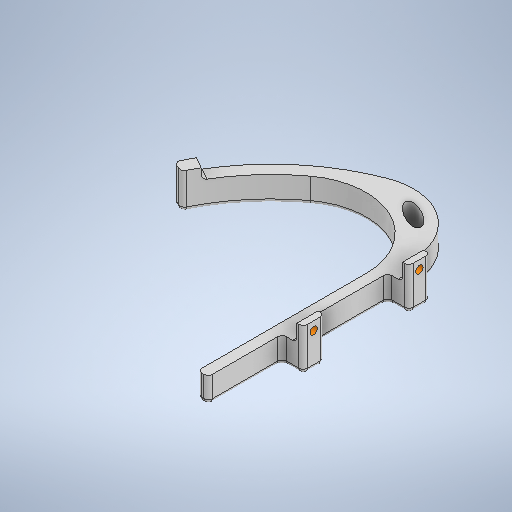
# Autodesk Inventor part: pare-chocs
Saved by Autodesk Inventor 2025 (Build 290162000, 162)
## iProperties
Created: 2024-10-10
Part Number: pare-chocs
Material: Générique
Document SubType Name: Modeling
Designer: chass
Density: 1 g/cm^3
Appearance: Par défaut
Author: chass
## iProperties of the stored document pare-chocs_Impression 3D.ipt
Created: 2025-01-09
Part Number: pare-chocs_Impression 3D
Material: Générique
Document SubType Name: Modeling
Designer: chass
Density: 1 g/cm^3
Appearance: Par défaut
Author: chass
Autodesk Inventor part; units mm, degrees
ref_plane "YZ Plane" through (0, 0, 0) normal (1, 0, 0) x (0, 1, 0)
ref_plane "XZ Plane" through (0, 0, 0) normal (0, 1, 0) x (-1, 0, 0)
ref_plane "XY Plane" through (0, 0, 0) normal (0, 0, 1) x (1, 0, 0)
sketch "Esquisse1" plane through (0, 0, 0) normal (1, 0, 0) x (0, 1, 0)
  line L0 (-2.5, 65) -> (2.5, 65)
  line L1 (2.5, 65) -> (2.5, -65)
  line L2 (2.5, -65) -> (-2.5, -65)
  line L3 (-2.5, -65) -> (-2.5, 65)
  line L4 (2.5, 65) -> (-2.5, -65)
  line L5 (2.5, -65) -> (-2.5, 65)
  point P0 (0, 0)
  point P1 (0, 0)
  point P2 (0, 0)
  dimension "d0" = 130
  dimension "d1" = 5
  constraints: 12 end point, 2 midpoint, 2 parallel, 1 coincident, 1 horizontal, 1 perpendicular
  measures "d0" distance of L0.end L1.end
  measures "d1" distance of L1.end L2.end
extrude "Extrusion1" add sketch "Esquisse1" along normal blind 5
sketch "Esquisse2" plane through (5, 0, 0) normal (1, 0, 0) x (0, 0, -1)
  line L0 (65, 2.5) -> (-65, 2.5) projected
  line L1 (-65, -2.5) -> (65, -2.5) projected
  line L2 (-30, 2.5) -> (-20, 2.5)
  line L3 (-20, 2.5) -> (-20, -2.5)
  line L4 (-20, -2.5) -> (-30, -2.5)
  line L5 (-30, -2.5) -> (-30, 2.5)
  line L6 (0, 13) -> (0, -16)
  line L7 (30, 2.5) -> (20, 2.5)
  line L8 (20, 2.5) -> (20, -2.5)
  line L9 (20, -2.5) -> (30, -2.5)
  line L10 (30, -2.5) -> (30, 2.5)
  point P0 (0, 0)
  point P1 (-20, 2.5)
  point P2 (30, -2.5)
  point P3 (30, 2.5)
  point P4 (20, 2.5)
  point P5 (20, -2.5)
  dimension "d4" = 10
  dimension "d5" = 20
  constraints: 18 end point, 4 symmetric about line, 3 point on line, 2 parallel, 1 horizontal, 1 perpendicular, 1 vertical
  measures "d4" distance between parallel lines of L3 L5
  measures "d5" distance between parallel lines of L3 L6
extrude "Extrusion2" add sketch "Esquisse2" along normal blind 10 contours L10 L1 L8 L0 | L3 L1 L5 L0
sketch "Esquisse3" plane through (0, 2.5, 65) normal (0, 1, 0) x (1, 0, 0)
  line L0 (15, 45) -> (15, 35) projected
  line L1 (5, 45) -> (15, 45) projected
  line L2 (15, 35) -> (12, 35)
  line L3 (12, 35) -> (12, 45)
  line L4 (12, 45) -> (15, 45)
  line L5 (15, 45) -> (15, 35)
  line L6 (-9, 65) -> (24, 65)
  line L7 (15, 85) -> (15, 95)
  line L8 (15, 95) -> (12, 95)
  line L9 (12, 95) -> (12, 85)
  line L10 (12, 85) -> (15, 85)
  line L11 (15, 85) -> (15, 95)
  point P0 (0, 65)
  constraints: 20 end point, 5 symmetric about line, 2 horizontal, 2 parallel, 1 perpendicular, 1 point on line
extrude "Extrusion3" add sketch "Esquisse3" along normal blind 15
sketch "Esquisse4" plane through (15, 0, 0) normal (1, 0, 0) x (0, 0, -1)
  circle A0 centre (-25, 13.5) radius 1.75
  line L0 (0, 20) -> (0, -21)
  circle A1 centre (25, 13.5) radius 1.75
  line L1 (-30, 17.5) -> (-20, 17.5) projected
  line L2 (-20, -2.5) -> (-20, 17.5) projected
  point P0 (0, 0)
  dimension "d10" = 3.5
  dimension "d11" = 4
  dimension "d19" = 5
  constraints: 2 centre point, 2 end point, 1 symmetric about line, 1 vertical, 1 other
  measures "d10" diameter of A0
  measures "d11" distance from line of L1 A0.centre
  measures "d19" distance from line of L2 A0.centre
extrude "Extrusion4" cut sketch "Esquisse4" against normal blind 10
sketch "Esquisse19" plane through (0, 2.5, 65) normal (0, 1, 0) x (1, 0, 0)
  line L0 (5, 130) -> (5, 95) projected
  line L1 (5, 130) -> (0, 130)
  line L2 (0, 130) -> (0, 0)
  line L3 (0, 0) -> (5, 0)
  line L4 (5, 0) -> (5, 130)
  point P0 (0, 65)
  constraints: 8 end point, 2 parallel, 1 horizontal, 1 perpendicular
extrude "Extrusion15" add sketch "Esquisse19" along normal blind 7
sketch "Esquisse21" plane through (0, -2.5, -65) normal (0, -1, 0) x (1, 0, 0)
  line L0 (0, 0) -> (0, 130) projected
  arc A0 (-86.0635, 54.7747) -> (0, 0) centre (0, 95) ccw
  arc A1 (-80.6279, 57.3152) -> (0, 6) centre (0, 95) ccw
  line L1 (-80.6279, 57.3152) -> (-86.0635, 54.7747)
  point P0 (0, 65)
  constraints: 4 point on circle, 2 centre point, 2 end point, 2 point on line, 1 coincident
extrude "Extrusion16" add sketch "Esquisse21" against normal blind 12
fillet "Congé18" radius 33.25 1 edges at (0, 3.5, -59)
fillet "Congé21" radius 28.5 1 edges at (5, 3.5, -65)
sketch "Esquisse22" plane through (5, 2.5, -20) normal (0, 1, 0) x (1, 0, 0)
  line L0 (0, 10) -> (10, 10) projected
  line L1 (0, 10) -> (7, 10)
  line L2 (7, 10) -> (7, 0)
  line L3 (7, 0) -> (0, 0)
  line L4 (0, 0) -> (0, 10)
  line L5 (0, -40) -> (10, -40) projected
  line L6 (0, -40) -> (7, -40)
  line L7 (7, -40) -> (7, -50)
  line L8 (7, -50) -> (0, -50)
  line L9 (0, -50) -> (0, -40)
  point P0 (-5, -20)
  constraints: 16 end point, 4 parallel, 2 horizontal, 2 perpendicular, 1 point on line
extrude "Extrusion17" add sketch "Esquisse22" along normal blind 7
fillet "Congé22" radius 2 2 edges at (12, 9.5, -25) (12, 9.5, 25)
fillet "Congé23" radius 2 6 edges at (5, 3.5, 30) (5, 3.5, 20) (5, 3.5, -20) (5, 3.5, -30) (15, -2.5, -25) (15, -2.5, 25)
fillet "Congé24" radius 2 2 edges at (0, 3.5, 65) (5, 3.5, 65)
sketch "Esquisse23" plane through (0, 9.5, 65) normal (0, 1, 0) x (1, 0, 0)
  ellipse E0 centre (-13, 115) end of major axis (-6.1401, 110.884) minor radius 3.0984
  point P0 (0, 65)
  dimension "d76" = 8
  constraints: 1 centre point
extrude "Extrusion18" cut sketch "Esquisse23" against normal blind 18.5
sketch "Esquisse24" plane through (0, 9.5, 65) normal (0, 1, 0) x (1, 0, 0)
  arc A0 (-33.5714, 123.8705) -> (-86.0635, 75.2253) centre (0, 35) ccw projected
  line L0 (-86.0635, 75.2253) -> (-80.6279, 72.6848) projected
  arc A1 (-82.5591, 82) -> (-86.0635, 75.2253) centre (0, 35) ccw
  arc A2 (-77.3448, 79.0316) -> (-80.6279, 72.6848) centre (0, 35) ccw
  line L1 (-77.3448, 79.0316) -> (-82.5591, 82)
  point P0 (0, 65)
  constraints: 5 point on circle, 2 centre point, 2 coincident, 2 end point
extrude "Extrusion19" add sketch "Esquisse24" along normal blind 5
fillet "Congé25" radius 2 3 edges at (-79.9519, 9.5, -15.5158) (-80.6279, 6, -7.6848) (-86.0635, 6, -10.2253)
fillet "Congé26" radius 2 30 edges at (14.4142, -1.9142, 30) (10, -2.5, 30) (5.5858, -2.5, 30.5858) (5, -2.5, 47.5) (4.4142, -2.5, 64.4142) (2.5, -2.5, 65) (0.5858, -2.5, 64.4142) (0, -2.5, 24.1253) (-18.3136, -2.5, -44.4556) (-68.329, -2.5, -27.0276) (-80.9113, -2.5, -8.4468) (-83.326, -2.5, -8.9458) (-85.2725, -2.5, -10.5191) (-63.8203, -2.5, -40.3702) (-7.2949, -2.5, -55.6538) (5, -2.5, -32.1047) (5.5858, -2.5, -30.5858) (10, -2.5, -30) (14.4142, -1.9142, -30) (15, 8.5, -30) (15, 8.5, 30) (14.4142, -1.9142, 20) (10, -2.5, 20) (5.5858, -2.5, 19.4142) (5, -2.5, 0) (5.5858, -2.5, -19.4142) (10, -2.5, -20) (14.4142, -1.9142, -20) (15, 8.5, -20) (15, 8.5, 20)
